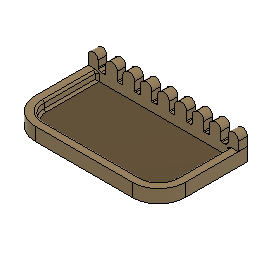
brush holder (Autodesk Fusion 360 design; units mm, degrees)
part number: 2026-07-21-01-10-24-036
Autodesk Fusion 360 part; units mm, degrees
note: some values were not read from the file. Chosen so that the rebuilt part matches the saved one: a direction; which pieces of a blend or face edit are solid.
sketch "Sketch1" plane through (0, 0, 0) normal (0, 1, 0) x (1, 0, 0)
  line L0 (110, -80) -> (-110, -80)
  line L1 (-150, -40) -> (-150, 80)
  line L2 (-150, 80) -> (150, 80)
  line L3 (150, 80) -> (150, -40)
  line L4 (150, -80) -> (-150, 80) construction
  line L5 (-150, -80) -> (150, 80) construction
  arc A0 (-150, -40) -> (-110, -80) centre (-110, -40) ccw
  arc A1 (110, -80) -> (150, -40) centre (110, -40) ccw
  arc A2 (-170, -40) -> (-110, -100) centre (-110, -40) ccw
  line L6 (110, -100) -> (-110, -100)
  arc A3 (110, -100) -> (170, -40) centre (110, -40) ccw
  line L7 (170, 100) -> (170, -40)
  line L8 (-170, 100) -> (170, 100)
  line L9 (-170, -40) -> (-170, 100)
  dimension "d1" = 40
  dimension "d2" = -20
  constraint horizontal L0
  constraint perpendicular L0 L1
  constraint parallel L0 L2
  constraint parallel L1 L3
  constraint coincident L4 origin
  constraint coincident L5 origin
  constraint coincident L5.start L0
  constraint coincident L5.start L1
  constraint tangent L0 A0
  constraint tangent L1 A0
  constraint coincident L4.start L0
  constraint coincident L4.start L3
  constraint tangent L0 A1
  constraint tangent L3 A1
  constraint equal A0 A1
  measures "d1" radius of A0
ref_plane "WorkPlane1" through (0, 0, -100) normal (0, 0, 1) x (1, 0, 0)
sketch "Sketch2" plane through (0, 0, -100) normal (0, 0, 1) x (1, 0, 0)
  line L0 (-170, 0) -> (-170, 50.631)
  line L1 (-170, 0) -> (170, 0)
  line L2 (-147.8843, 50.5431) -> (-147.8719, 35.876)
  arc A0 (-147.8843, 50.5431) -> (-170, 50.631) centre (-158.9424, 50.5338) ccw
  arc A1 (-147.1119, 33.7902) -> (-128.5888, 33.6964) centre (-137.8106, 41.5917) ccw
  line L3 (-127.8076, 50.6313) -> (-127.8076, 35.8101)
  line L4 (-127.8075, 0) -> (-104.6017, 0)
  line L5 (-104.6017, 49.841) -> (-104.6017, 0)
  arc A2 (-104.6017, 49.841) -> (-127.8076, 50.6313) centre (-116.1638, 51.4334) ccw
  arc A3 (-147.8719, 35.876) -> (-147.1119, 33.7902) centre (-144.6219, 35.8788) ccw
  arc A4 (-128.5888, 33.6964) -> (-127.8076, 35.8101) centre (-131.0576, 35.8101) ccw
  line L6 (-127.8075, 0) -> (-170, 0)
  point P0 (-170, 0)
  dimension "d4" = 3.25
  constraint coincident P0 L0.start
  constraint tangent L2 A0
  constraint coincident L1 L4.start
  constraint perpendicular L1 L3
  constraint coincident L1 L4.end
  constraint perpendicular L4 L5
  constraint tangent L2 A3
  constraint tangent A1 A3
  constraint tangent A1 A4
  constraint tangent L3 A4
  constraint equal A3 A4
  constraint perpendicular L0 L6
  measures "d4" radius of A3
extrude "Extrude1" add sketch "Sketch2" along normal blind 20 makes body 1
pattern_path "PathPattern1" count 8 spacing 39.217 from (-137.2463, 0, -80) backwards path "Sketch1" along A1 L0 A0 L1 L2 L3 of bodies 1 makes body 2 at (-107.163, 9.9913, -100) makes body 3 at (-91.5661, 16.877, -93.3333) makes body 4 at (-52.3491, 16.877, -93.3333) makes body 5 at (-13.1321, 16.877, -93.3333) makes body 6 at (26.0849, 16.877, -93.3333) makes body 7 at (65.3018, 16.877, -93.3333) makes body 8 at (104.5188, 16.877, -93.3333)
extrude "Extrude2" add sketch "Sketch1" along normal blind 10 contours L0 L1 L2 L3 A0 A1 bodies 1 2 3 4 5 6 7 8
extrude "Extrude3" add sketch "Sketch1" along normal blind 30 bodies 1
fillet "Fillet1" radius 4.5 5 faces at (36.6667, 16.6667, 80) (-128.3291, 23.3333, 75.5534) (-150, 16.6667, 0) (147.8, 23.3333, 53.0827) (150, 16.6667, -40) on bodies 1
scale "Scale1" factor 0.27 about (110, 10, 75.5) bodies 1
move_body "Move1" bodies 1 to x (1, 0, 0) y (0, 1, 0) z (0, 0, 1) at (-80.3, -10, -54.5075)
named bodies: "main"
